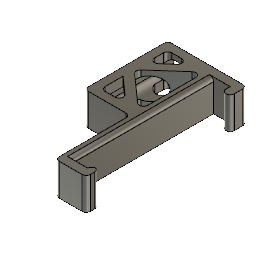
y_Axis_ScreHolder (Autodesk Fusion 360 design; units mm, degrees)
Autodesk Fusion 360 part; units mm, degrees
sketch "Sketch1" plane through (0, 0, 0) normal (0, 0, 1) x (1, 0, 0)
  line L0 (20.9846, 55.2598) -> (20.9846, 21.2598)
  line L1 (20.9846, 55.2598) -> (24.9846, 55.2598)
  line L2 (24.9846, 55.2598) -> (24.9846, 53.2598)
  line L3 (24.9846, 53.2598) -> (26.9846, 53.2598)
  line L4 (26.9846, 53.2598) -> (26.9846, 57.2598)
  line L5 (26.9846, 57.2598) -> (7.9846, 57.2598)
  line L6 (7.9846, 57.2598) -> (7.9846, 37.2598)
  line L7 (7.9846, 37.2598) -> (18.9846, 37.2598)
  line L8 (18.9846, 37.2598) -> (18.9846, 19.2598)
  line L9 (18.9846, 19.2598) -> (26.485, 19.2598)
  line L10 (20.9846, 21.2598) -> (24.6846, 21.2598)
  line L11 (24.6846, 21.2598) -> (25.485, 22.2598)
  line L12 (25.485, 22.2598) -> (26.485, 22.2598)
  line L13 (26.485, 22.2598) -> (26.485, 19.2598)
  line L14 (9.9846, 55.2598) -> (15.9742, 55.2598)
  line L15 (15.9742, 55.2598) -> (9.9846, 49.9357)
  line L16 (9.9846, 49.9357) -> (9.9846, 55.2598)
  line L17 (9.9846, 44.5839) -> (9.9846, 39.2598)
  line L18 (9.9846, 39.2598) -> (15.9742, 39.2598)
  line L19 (9.9846, 44.5839) -> (15.9742, 39.2598)
  line L20 (9.9846, 47.2598) -> (18.9846, 55.2598)
  line L21 (18.9846, 39.2598) -> (9.9846, 47.2598)
  line L22 (18.9846, 39.2598) -> (18.9846, 55.2598)
  dimension "d1" = 2
  dimension "d2" = 4
  dimension "d3" = 2
  dimension "d4" = 2
  dimension "d5" = 13
  dimension "d6" = 34
  dimension "d7" = 1
  dimension "d8" = 3.7
  dimension "d9" = 1
  dimension "d10" = 2
  dimension "d11" = 20
  dimension "d15" = 2
  dimension "d25" = 2
  dimension "d26" = 2
  dimension "d27" = 2
  dimension "d29" = 2
  dimension "d30" = 2
  dimension "d31" = 2
  dimension "d32" = 2
  dimension "d34" = 2
  dimension "d35" = 2
  constraint vertical L0
  constraint perpendicular L0 L1
  constraint perpendicular L1 L2
  constraint perpendicular L2 L3
  constraint perpendicular L3 L4
  constraint perpendicular L4 L5
  constraint perpendicular L5 L6
  constraint perpendicular L6 L7
  constraint perpendicular L7 L8
  constraint perpendicular L8 L9
  constraint perpendicular L0 L10
  constraint perpendicular L0 L12
  constraint perpendicular L9 L13
  constraint horizontal L14
  constraint perpendicular L14 L16
  constraint perpendicular L14 L17
  constraint perpendicular L17 L18
  constraint perpendicular L18 L22
  constraint parallel L15 L20
  constraint parallel L19 L21
  constraint equal L16 L17
  constraint equal L14 L18
  measures "d1" distance of L0 L8
  measures "d2" distance of L0.start L1.end
  measures "d3" distance of L2 L4
  measures "d4" distance of L1.end L2.end
  measures "d5" distance of L0 L6
  measures "d6" distance of L0.start L0.end
  measures "d7" distance of L11.end L12.end
  measures "d8" distance of L0.end L10.end
  measures "d9" distance of L10 L12
  measures "d10" distance of L9 L10
  measures "d11" distance of L5 L7
  measures "d15" distance of L1 L5
  measures "d25" distance of L6 L16
  measures "d26" distance of L19 L21
  measures "d27" distance of L0 L22
  measures "d29" distance of L15 L20
  measures "d30" distance of L5 L14
  measures "d31" distance of L6 L17
  measures "d32" distance of L7 L18
  measures "d34" distance of L6 L20.start
  measures "d35" distance of L7 L21.start
extrude "Extrude1" add sketch "Sketch1" along normal blind 7.7
fillet "Fillet1" radius 1 9 edges at (7.9846, 37.2598, 3.85) (18.9846, 37.2598, 3.85) (18.9846, 19.2598, 3.85) (26.485, 19.2598, 3.85) (7.9846, 57.2598, 3.85) (26.485, 22.2598, 3.85) (24.9846, 53.2598, 3.85) (26.9846, 53.2598, 3.85) (26.9846, 57.2598, 3.85)
fillet "Fillet1" radius 1 9 edges at (9.9846, 55.2598, 3.85) (15.9742, 55.2598, 3.85) (15.9742, 39.2598, 3.85) (9.9846, 39.2598, 3.85) (20.9846, 38.2598, 7.7) (9.9846, 49.9357, 3.85) (9.9846, 47.2598, 3.85) (18.9846, 55.2598, 3.85) (18.9846, 39.2598, 3.85)
sketch "Sketch2" plane through (0, 57.2598, 0) normal (0, 1, 0) x (-1, 0, 0)
  line L0 (-25.9846, 7.7) -> (-25.9846, 0)
  line L1 (-25.9846, 0) -> (-8.9846, 0)
  line L2 (-8.9846, 0) -> (-8.9846, 7.7)
  line L3 (-8.9846, 7.7) -> (-25.9846, 7.7)
  line L4 (-26.9846, 7.7) -> (-26.9846, 0)
  line L5 (-7.9846, 0) -> (-7.9846, 7.7)
  line L6 (-20.9846, 0) -> (-20.9846, 6.7)
  point P0 (-11.9846, 4)
  point P1 (-20.9846, 0)
  point P2 (-11.9846, 3.7)
  dimension "d16" = 4
  dimension "d22" = 9
  dimension "d23" = 9
  dimension "d24" = 4
  measures "d16" distance of L1 P0
  measures "d22" horizontal distance of P0 P1
  measures "d23" distance of P2 L6
  measures "d24" distance of L3 P2
hole "Hole1" at (11.9846, 57.2598, 4) at (11.9846, 57.2598, 3.7) direction (0, -1, 0) diameter 5 depth 18 tip angle 160
